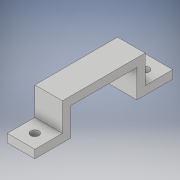
# Autodesk Inventor part: 000.210 - Скоба
Saved by Autodesk Inventor 2019 (Build 230136000, 136)
## iProperties
Created: 2020-04-11
Part Number: 000.210 - Скоба
Material: Типовые
Document SubType Name: Modeling
Designer: Петров Иван
Density: 1 g/cm^3
Appearance: По умолчанию
Author: Петров Иван
Autodesk Inventor part; units mm, degrees
ref_plane "YZ Plane" through (0, 0, 0) normal (1, 0, 0) x (0, 1, 0)
ref_plane "XZ Plane" through (0, 0, 0) normal (0, 1, 0) x (-1, 0, 0)
ref_plane "XY Plane" through (0, 0, 0) normal (0, 0, 1) x (1, 0, 0)
sketch "Эскиз1" plane through (0, 0, 0) normal (0, 1, 0) x (-1, 0, 0)
  line L0 (0, 0) -> (0, -12)
  line L1 (0, -12) -> (0, -20)
  line L2 (-5, -15) -> (5, -15)
  line L3 (5, -15) -> (5, -25)
  line L4 (5, -25) -> (-5, -25)
  line L5 (-5, -25) -> (-5, -15)
  line L6 (-5, -15) -> (5, -25) construction
  line L7 (5, -15) -> (-5, -25) construction
  circle A0 centre (0, -20) radius 1.5
  dimension "d0" = 12
  dimension "d1" = 8
  dimension "d2" = 10
  dimension "d3" = 10
  dimension "d4" = 3
  constraints: 16 end point, 2 midpoint, 2 parallel, 1 centre point, 1 coincident, 1 horizontal, 1 perpendicular, 1 point on line, 1 vertical
  measures "d0" distance of L0.start L0.end
  measures "d1" distance of L0.end L1.end
  measures "d2" distance of L3.end L4.end
  measures "d3" distance of L2.end L3.end
  measures "d4" diameter of A0
extrude "Выдавливание1" add sketch "Эскиз1" along normal blind 3
sketch "Эскиз2" plane through (0, 3, 0) normal (0, 1, 0) x (1, 0, 0)
  line L0 (-5, 15) -> (5, 15) projected
  line L1 (-5, 15) -> (5, 15)
  line L2 (5, 15) -> (5, 12)
  line L3 (5, 12) -> (-5, 12)
  line L4 (-5, 12) -> (-5, 15)
  point P0 (0, 0)
  dimension "d7" = 3
  constraints: 8 end point, 2 parallel, 1 horizontal, 1 perpendicular
  measures "d7" distance of L1.end L2.end
extrude "Выдавливание2" add sketch "Эскиз2" along normal blind 7.2 and the other way blind 3
sketch "Эскиз3" plane through (0, 10.2, 0) normal (0, 1, 0) x (1, 0, 0)
  line L0 (5, 15) -> (-5, 15) projected
  line L1 (5, 15) -> (-5, 15)
  line L2 (-5, 15) -> (-5, 0)
  line L3 (-5, 0) -> (5, 0)
  line L4 (5, 0) -> (5, 15)
  point P0 (0, 0)
  dimension "d12" = 10
  constraints: 8 end point, 2 parallel, 1 horizontal, 1 perpendicular
  measures "d12" distance of L3.end L2.end
extrude "Выдавливание3" add sketch "Эскиз3" along normal blind 3
mirror "Зеркальное отражение1" about plane through (0, 0, 0) normal (0, 0, 1) of "Выдавливание2", "Выдавливание3", "Выдавливание1"
